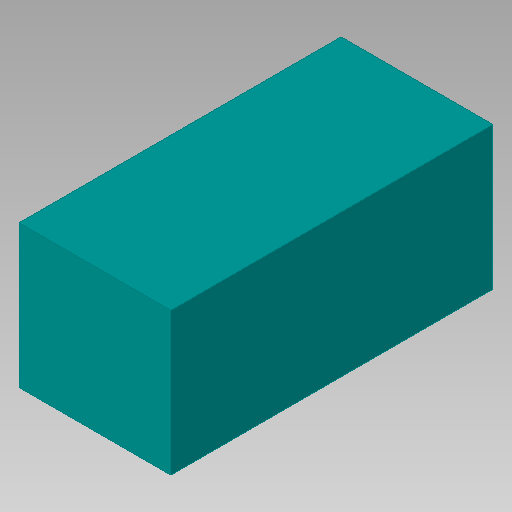
# Autodesk Inventor part: MS_TM
Saved by Autodesk Inventor 2020.1 (Build 241239000, 239)
## iProperties
Created: 2015-11-24
Part Number: MS_TM
Material: Generic
Document SubType Name: Modeling
Designer: PhillipD
Density: 1 g/cm^3
Appearance: MS_TM, MS_TM
Author: PhillipD
Autodesk Inventor part; units mm, degrees
ref_plane "YZ Plane" through (0, 0, 0) normal (1, 0, 0) x (0, 1, 0)
ref_plane "XZ Plane" through (0, 0, 0) normal (0, 1, 0) x (-1, 0, 0)
ref_plane "XY Plane" through (0, 0, 0) normal (0, 0, 1) x (1, 0, 0)
sketch "MS_TM, MS_TM_158" plane through (0, 0, 0) normal (0, 0, 1) x (1, 0, 0)
  line L0 (0, 0.4432) -> (0.4712, 0.4432)
  line L1 (0.4712, 0.4432) -> (0.4712, 0)
  line L2 (0.4712, 0) -> (0, 0)
  line L3 (0, 0) -> (0, 0.4432)
  constraints: 8 end point
extrude "Extrusion1" add sketch "MS_TM, MS_TM_158" along normal blind 1
body "Solid1"
